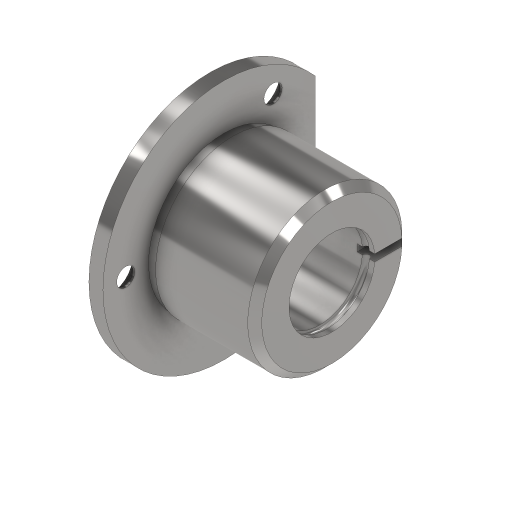
# Autodesk Inventor part: Part009Flange
Saved by Autodesk Inventor 2023.2 (Build 272271030, 271C)
## iProperties
Created: 2023-09-08
Part Number: Part009Flange
Material: Steel, Carbon
Document SubType Name: Modeling
Designer: User
Density: 7.85 g/cm^3
Appearance: Steel - Polished
Author: User
Autodesk Inventor part; units mm, degrees
ref_plane "YZ Plane" through (0, 0, 0) normal (1, 0, 0) x (0, 1, 0)
ref_plane "XZ Plane" through (0, 0, 0) normal (0, 1, 0) x (-1, 0, 0)
ref_plane "XY Plane" through (0, 0, 0) normal (0, 0, 1) x (1, 0, 0)
sketch "Sketch1" plane through (0, 0, 0) normal (0, 0, 1) x (1, 0, 0)
  line L0 (0, 34.5) -> (0, 12.25)
  line L1 (0, 12.25) -> (1.5, 12.25)
  line L2 (34.8, 12.25) -> (34.8, 22)
  line L3 (34.8, 22) -> (6.5, 22)
  line L4 (4, 21.5) -> (4, 34.5)
  line L5 (0, 34.5) -> (4, 34.5)
  line L6 (-6.96, 0) -> (41.76, 0) projected
  line L7 (6.5, 22) -> (6.5, 21.5)
  line L8 (6.5, 21.5) -> (4, 21.5)
  arc A0 (3.5, 12.25) -> (1.5, 12.25) centre (2.5, 12.25) ccw
  arc A1 (33.3, 12.25) -> (31.3, 12.25) centre (32.3, 12.25) ccw
  line L9 (1.5, 12.25) -> (3.5, 12.25) construction
  line L10 (3.5, 12.25) -> (31.3, 12.25)
  line L11 (31.3, 12.25) -> (33.3, 12.25) construction
  line L12 (33.3, 12.25) -> (34.8, 12.25)
  point P0 (0, 0)
  dimension "d0" = 34.8
  dimension "d1" = 69
  dimension "d2" = 24.5
  dimension "d3" = 44
  dimension "d4" = 4
  dimension "d5" = 43
  dimension "d6" = 2.5
  dimension "d7" = 1
  dimension "d8" = 1
  dimension "d9" = 2.5
  dimension "d10" = 2.5
  constraints: 24 end point, 12 perpendicular, 5 point on line, 4 point on circle, 3 vertical, 2 centre point, 2 midpoint, 1 horizontal
  measures "d0" distance of L0.end L2.start
  measures "d1" diameter of L5 L6
  measures "d2" diameter of L1 L6
  measures "d3" diameter of L3 L6
  measures "d4" distance of L0.start L4.end
  measures "d5" diameter of L8 L6
  measures "d6" distance of L7.end L4.start
  measures "d7" radius of A0
  measures "d8" radius of A1
  measures "d9" distance from line of L2 A1.centre
  measures "d10" distance from line of L0 A0.centre
revolve "Revolution1" add sketch "Sketch1" angle 360 about axis through (-10, 0, 0) along (1, 0, 0)
chamfer "Chamfer1" distance 2 angle 45 1 edges at (34.8, -22, 0)
sketch "Sketch2" plane through (0, 0, 0) normal (0, 0, 1) x (1, 0, 0)
  line L0 (34.8, -12.25) -> (34.8, 12.25) projected
  line L1 (34.8, 1) -> (29.8, 1)
  line L2 (29.8, 1) -> (29.8, -1)
  line L3 (29.8, -1) -> (34.8, -1)
  line L4 (34.8, -1) -> (34.8, 1)
  point P0 (0, 0)
  point P1 (34.8, 0)
  point P2 (29.8, 0)
  dimension "d15" = 2
  dimension "d16" = 5
  constraints: 8 end point, 3 midpoint, 2 parallel, 1 horizontal, 1 perpendicular
  measures "d15" distance between parallel lines of L3 L1
  measures "d16" distance from line of point (29.8, 0) L0
extrude "Extrusion1" cut sketch "Sketch2" against normal through all
sketch "Sketch3" plane through (0, 0, 0) normal (-1, 0, 0) x (0, 0, 1)
  circle A0 centre (0, 0) radius 12.25 projected
  point P0 (28, 0)
  dimension "d19" = 28
  constraints: 1 horizontal alignment
  measures "d19" distance of point (28, 0) A0.centre
hole "Hole1" at (0, 0, 28) direction (1, 0, 0) diameter 5.2 end through all countersink diameter 12 countersink angle 90
pattern_circular "Circular Pattern1" count 3 over 360 about axis through (2, 0, 0) along (1, 0, 0) of "Hole1"
sketch "Sketch4" plane through (0, 0, 0) normal (-1, 0, 0) x (0, 0, 1)
  circle A0 centre (0, 0) radius 12.25 projected
  circle A1 centre (0, 0) radius 34.5 projected
  line L0 (-26, 22.6771) -> (-26, -22.6771)
  dimension "d30" = 26
  constraints: 2 end point, 2 point on circle, 1 vertical
  measures "d30" distance from line of L0 A0.centre
extrude "Extrusion2" cut sketch "Sketch4" against normal through all contours L0 A1 picked at (-27.5435, 5.2917)
body "Solid1"
